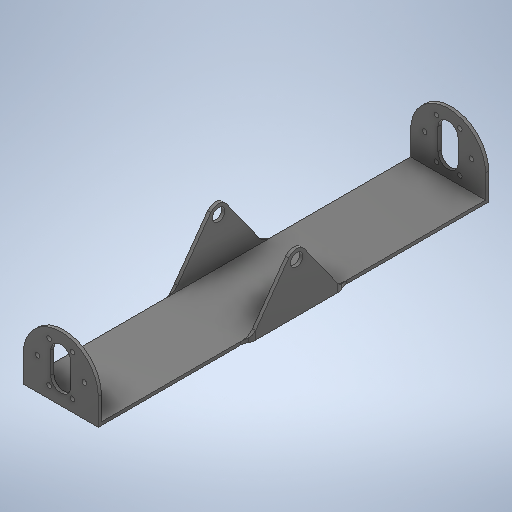
# Autodesk Inventor part: 520 DC Pendulum Bottom Bracket
Saved by Autodesk Inventor 2025.2 (Build 292293000, 293)
## iProperties
Created: 2025-01-23
Part Number: 520 DC Pendulum Bottom Bracket
Material: Generic
Document SubType Name: Modeling
Designer: Matt Tidd
Density: 1 g/cm^3
Appearance: Default
Mass: 29.0631 g
Surface Area: 310.336 cm^2
Volume: 29.0631 cm^3
Author: Matt Tidd
Autodesk Inventor part; units mm, degrees
ref_plane "YZ Plane" through (0, 0, 0) normal (1, 0, 0) x (0, 1, 0)
ref_plane "XZ Plane" through (0, 0, 0) normal (0, 1, 0) x (-1, 0, 0)
ref_plane "XY Plane" through (0, 0, 0) normal (0, 0, 1) x (1, 0, 0)
sketch "Sketch1" plane through (0, 0, 0) normal (0, 1, 0) x (-1, 0, 0)
  line L0 (0, 0) -> (48, 0)
  line L1 (48, 0) -> (48, -250)
  line L2 (48, -250) -> (0, -250)
  line L3 (0, -250) -> (0, 0)
  dimension "d0" = 48
  dimension "d1" = 250
  constraints: 8 end point, 2 parallel, 1 horizontal, 1 perpendicular
  measures "d0" distance of L1.end L2.end
  measures "d1" distance of L0.end L1.end
extrude "Extrusion1" add sketch "Sketch1" along normal blind 2
sketch "Sketch2" plane through (-48, 0, 0) normal (0, 0, 1) x (1, 0, 0)
  line L0 (48, 2) -> (0, 2) projected
  line L1 (0, 2) -> (44, 2)
  line L2 (0, 2) -> (48, 2)
  line L3 (48, 2) -> (48, 41)
  line L4 (48, 41) -> (0, 41)
  line L5 (0, 41) -> (0, 2)
  arc A0 (48, 17) -> (0, 17) centre (24, 17) ccw
  line L6 (48, 17) -> (0, 17) construction
  line L7 (48, 17) -> (96, 17) construction
  line L8 (24, 27.5) -> (24, 13.5) construction
  line L9 (17.5, 27.5) -> (17.5, 13.5)
  line L10 (30.5, 13.5) -> (30.5, 27.5)
  arc A1 (30.5, 27.5) -> (17.5, 27.5) centre (24, 27.5) ccw
  arc A2 (17.5, 13.5) -> (30.5, 13.5) centre (24, 13.5) ccw
  line L11 (24, 27.5) -> (38, 27.5) construction
  circle A3 centre (39, 20.5) radius 1.5
  circle A4 centre (31.5, 33.4904) radius 1.5
  circle A5 centre (16.5, 33.4904) radius 1.5
  circle A6 centre (9, 20.5) radius 1.5
  circle A7 centre (16.5, 7.5096) radius 1.5
  circle A8 centre (31.5, 7.5096) radius 1.5
  point P0 (24, 20.5)
  point P1 (24, 20.5)
  point P2 (48, 2)
  dimension "d77" = 48
  dimension "d78" = 39
  dimension "d79" = 180
  dimension "d80" = 14
  dimension "d81" = 90
  dimension "d82" = 13
  dimension "d83" = 3
  dimension "d86" = 360
  constraints: 24 end point, 9 centre point, 6 point on circle, 6 tangent, 4 horizontal, 3 parallel, 2 equal length, 2 perpendicular, 2 point on line, 1 midpoint, 13 other
  measures "d77" distance of L4.end L3.end
  measures "d78" distance of L3.end L2.end
  measures "d79" angle of L6 L7
  measures "d80" distance of L8.start L8.end
  measures "d81" angle of L8 L11
  measures "d82" diameter of A2
  measures "d83" diameter of A3
extrude "Extrusion2" add sketch "Sketch2" against normal blind 2 contours L0 L5 A0 L3
sketch "Sketch5" plane through (0, 0, 0) normal (1, 0, 0) x (0, 0, -1)
  line L0 (250, 2) -> (2, 2) construction
  line L1 (130, 2) -> (193.1782, 2) construction
  line L2 (130, 0) -> (184.309, 0) construction
  line L3 (250, 0) -> (0, 0) projected
  line L4 (125, 2) -> (125, 0) construction
  line L5 (95, 0) -> (155, 0)
  line L6 (155, 0) -> (155, 2)
  line L7 (155, 2) -> (95, 2)
  line L8 (95, 2) -> (95, 0)
  circle A0 centre (125, 31.4375) radius 4
  circle A1 centre (125, 31.4375) radius 6.125
  line L9 (155, 0) -> (129.9829, 34.9992)
  line L10 (95, 0) -> (120.0171, 34.9992)
  line L11 (96.4296, 2) -> (96.4296, 0)
  line L12 (153.5704, 2) -> (153.5704, 0)
  point P0 (0, 2)
  dimension "d91" = 60
  dimension "d92" = 2
  dimension "d93" = 8
  dimension "d94" = 12.25
  constraints: 22 end point, 8 point on line, 3 horizontal, 3 perpendicular, 2 centre point, 2 parallel, 2 point on circle, 2 tangent, 1 coincident, 1 midpoint
  measures "d91" distance of L7.end L6.end
  measures "d92" distance of L6.end L5.end
  measures "d93" diameter of A0
  measures "d94" diameter of A1
extrude "Extrusion4" add sketch "Sketch5" along normal blind 2 contours L3 L11 L7 L12 | L7 L10 A1 L9 | A1
sketch "Sketch6" plane through (0, 2, 0) normal (0, 1, 0) x (1, 0, 0)
  line L0 (0, 250) -> (-48, 250) construction
  line L1 (-24, 250) -> (-24, 50) construction
  line L2 (-48, 250) -> (-48, 0) construction
  line L3 (-48, 125) -> (0, 125) construction
  line L4 (0, 128.5704) -> (0, 104.9829) construction
  point P0 (0, 0)
  point P1 (-48, 2)
  constraints: 4 end point, 2 midpoint, 1 horizontal, 1 point on line, 1 vertical
ref_plane "Work Plane5" through (-24, 2, -250) normal (-1, 0, 0) x (0, 0, 1)
ref_plane "Work Plane6" through (-48, 2, -125) normal (0, 0, 1) x (1, 0, 0)
mirror "Mirror5" about plane through (-24, 2, -250) normal (-1, 0, 0) of "Extrusion4"
mirror "Mirror6" about plane through (-48, 2, -125) normal (0, 0, 1) of "Extrusion2"
fillet "Fillet12" radius 8 4 edges at (0, 1, -96.4296) (0, 1, -153.5704) (-48, 1, -153.5704) (-48, 1, -96.4296)
fillet "Fillet13" radius 8 4 edges at (-48.92, 2, -96.4296) (-48.92, 2, -153.5704) (0.92, 2, -153.5704) (0.92, 2, -96.4296)
fillet "Fillet14" radius 8 4 edges at (2, 1.5698, -96.4296) (2, 1.5698, -153.5704) (-50, 1.5698, -153.5704) (-50, 1.5698, -96.4296)
body "Solid1"
